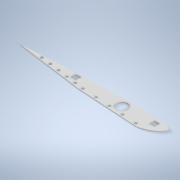
# Autodesk Inventor part: airfoil
Saved by Autodesk Inventor 2021 (Build 250183000, 183)
## iProperties
Created: 2021-03-04
Part Number: airfoil
Material: Generic
Document SubType Name: Modeling
Designer: Ferdinand Hubbard
Density: 1 g/cm^3
Appearance: Default
Author: Ferdinand Hubbard
Autodesk Inventor part; units mm, degrees
ref_plane "YZ Plane" through (0, 0, 0) normal (1, 0, 0) x (0, 1, 0)
ref_plane "XZ Plane" through (0, 0, 0) normal (0, 1, 0) x (-1, 0, 0)
ref_plane "XY Plane" through (0, 0, 0) normal (0, 0, 1) x (1, 0, 0)
sketch "Sketch1" plane through (0, 0, 0) normal (0, 1, 0) x (-1, 0, 0)
  circle A0 centre (105.5716, 8.1262) radius 14.25
  circle A1 centre (105.5716, 8.1262) radius 9.25
  line L0 (22.2, 11.4019) -> (35.2, 11.4019)
  line L1 (35.2, 11.4019) -> (35.2, -1.5981)
  line L2 (35.2, -1.5981) -> (22.2, -1.5981)
  line L3 (22.2, -1.5981) -> (22.2, 11.4019)
  line L4 (218.3762, 9.117) -> (231.3762, 9.117)
  line L5 (231.3762, 9.117) -> (231.3762, -3.883)
  line L6 (231.3762, -3.883) -> (218.3762, -3.883)
  line L7 (218.3762, -3.883) -> (218.3762, 9.117)
  circle A2 centre (364, -0.1617) radius 156.5 construction
  circle A3 centre (201.1292, 22.785) radius 156.5 construction
  line L8 (45.2771, 32.5319) -> (201.1292, 22.785)
  line L9 (363.0659, -0.0318) -> (208.9905, 21.3865)
  circle A4 centre (53.4178, 26.5131) radius 3.5
  circle A5 centre (88.1392, 24.3452) radius 3.5
  circle A6 centre (122.8606, 22.1774) radius 3.5
  circle A7 centre (157.582, 20.0096) radius 3.5
  circle A8 centre (192.3034, 17.8418) radius 3.5
  circle A9 centre (308.9407, 1.9393) radius 3.5
  line L10 (244.7644, 10.8606) -> (145.7169, 24.6294) construction
  line L11 (244.7644, 10.8606) -> (343.8179, -2.909) construction
  line L12 (208.9905, 21.3865) -> (214.4381, 20.6292) construction
  line L13 (308.9407, 1.9393) -> (309.698, 7.387) construction
  line L14 (214.4381, 20.6292) -> (238.2531, 17.3187) construction
  line L15 (238.2531, 17.3187) -> (262.0681, 14.0081) construction
  line L16 (262.0681, 14.0081) -> (285.8831, 10.6975) construction
  line L17 (285.8831, 10.6975) -> (309.6981, 7.3869) construction
  line L18 (214.4381, 20.6292) -> (213.6809, 15.1816) construction
  line L19 (238.2531, 17.3187) -> (237.4959, 11.871) construction
  circle A10 centre (213.6809, 15.1816) radius 3.5
  circle A11 centre (237.4959, 11.871) radius 3.5
  line L20 (262.0681, 14.0081) -> (261.3108, 8.5605) construction
  line L21 (285.8831, 10.6975) -> (285.1258, 5.2499) construction
  circle A12 centre (261.3108, 8.5605) radius 3.5
  circle A13 centre (285.1258, 5.2499) radius 3.5
  spline S0 degree 4 poles (45.2771, 32.5319) (41.5409, 31.6235) (35.6173, 29.7503) (27.9433, 26.9303) (19.3063, 22.5208) (12.8749, 18.2077) (7.7345, 14.0731) (3.8722, 9.2552) (1.4864, 6.2872) (0.043, 1.3745) (-0.0312, 0.3812) (0.0281, -0.8778) (0.1745, -1.4612) (0.3929, -2.0102) (0.8084, -2.4627) (1.3186, -2.8975) (2.6239, -3.7046) (3.653, -4.1929) (10.4393, -6.6384) (15.6655, -7.3545) (25.1, -8.9784) (35.2344, -9.7015) (47.6639, -10.3746) (61.4155, -10.6998) (76.7019, -10.8882) (93.186, -10.8841) (110.736, -10.7454) (129.1149, -10.4736) (148.1138, -10.0951) (167.5031, -9.6193) (187.0543, -9.0657) (206.5356, -8.4416) (225.7153, -7.7631) (244.3709, -7.0324) (262.2765, -6.2607) (279.2509, -5.4328) (295.0539, -4.5223) (309.7119, -3.5525) (322.672, -2.6096) (334.6864, -1.7311) (343.575, -1.0514) (353.0562, -0.487) (356.1651, -0.2567) (362.8735, -0.0152) (362.7416, -0.02) (363.0659, -0.0318) knots 0 0 0 0 0 0.037834 0.062048 0.085007 0.106643 0.126842 0.145458 0.16091 0.173408 0.182937 0.189909 0.196272 0.202293 0.208895 0.216296 0.226837 0.241196 0.259494 0.282121 0.307217 0.334444 0.363559 0.394326 0.426495 0.459817 0.494058 0.528992 0.564399 0.600063 0.635772 0.671312 0.706467 0.741023 0.774768 0.8075 0.839017 0.869102 0.897496 0.923869 0.947785 0.968629 0.984176 1 1 1 1 1
  spline S1 degree 4 poles (208.9905, 21.3865) (207.0256, 21.743) (205.0603, 22.0965) (203.0947, 22.444) (201.1292, 22.785) knots 0.200177 0.200177 0.200177 0.200177 0.200177 0.208976 0.208976 0.208976 0.208976 0.208976
  point P0 (0, 0)
  point P1 (359.0762, 0.1364)
  point P2 (352.983, 0.4477)
  point P3 (344.5923, 1.0476)
  point P4 (334.0615, 2.0094)
  point P5 (321.589, 3.3822)
  point P6 (307.4061, 5.186)
  point P7 (291.7666, 7.4112)
  point P8 (274.9383, 10.0199)
  point P9 (257.194, 12.9452)
  point P10 (238.8043, 16.1074)
  point P11 (220.0304, 19.3803)
  point P12 (182.3116, 25.884)
  point P13 (163.8086, 28.8383)
  point P14 (145.8054, 31.4519)
  point P15 (128.4709, 33.6056)
  point P16 (111.9535, 35.2083)
  point P17 (96.3823, 36.1751)
  point P18 (81.868, 36.4427)
  point P19 (68.5109, 35.9373)
  point P20 (56.3246, 34.585)
  point P21 (26.5856, 26.0467)
  point P22 (18.9844, 22.098)
  point P23 (12.6078, 17.8447)
  point P24 (7.5002, 13.4274)
  point P25 (3.6892, 9.0035)
  point P26 (1.1921, 4.7745)
  point P27 (0.0659, 1.0017)
  point P28 (0.0006, -0.063)
  point P29 (0.0749, -0.9695)
  point P30 (0.2078, -1.5106)
  point P31 (0.424, -1.9791)
  point P32 (0.7616, -2.3945)
  point P33 (1.2282, -2.7955)
  point P34 (2.1216, -3.3822)
  point P35 (3.2232, -3.9537)
  point P36 (8.1428, -5.7128)
  point P37 (15.1176, -7.3056)
  point P38 (23.9224, -8.6283)
  point P39 (34.4841, -9.6094)
  point P40 (46.7728, -10.2571)
  point P41 (60.6811, -10.6511)
  point P42 (76.0314, -10.8426)
  point P43 (92.6351, -10.8589)
  point P44 (110.2911, -10.7246)
  point P45 (128.7881, -10.4591)
  point P46 (147.9055, -10.0812)
  point P47 (167.4164, -9.6062)
  point P48 (187.0898, -9.0495)
  point P49 (206.6927, -8.4228)
  point P50 (225.993, -7.7378)
  point P51 (244.7618, -7.0012)
  point P52 (262.7756, -6.217)
  point P53 (279.8246, -5.3721)
  point P54 (295.7441, -4.4524)
  point P55 (310.4019, -3.4858)
  point P56 (323.6531, -2.5368)
  point P57 (335.3351, -1.6764)
  point P58 (345.271, -0.9701)
  point P59 (353.2753, -0.4606)
  point P60 (359.1655, -0.1576)
  point P61 (362.7814, -0.0252)
  dimension "d2" = 28.5
  dimension "d3" = 18.5
  dimension "d12" = 13
  dimension "d13" = 13
  dimension "d14" = 13
  dimension "d15" = 13
  dimension "d44" = 7
  dimension "d45" = 7
  dimension "d48" = 7
  dimension "d49" = 47.3016
  dimension "d50" = 7
  dimension "d62" = 5.5
  dimension "d71" = 156.1566
  dimension "d72" = 155.557
  constraints: 44 end point, 13 centre point, 11 point on line, 6 coincident, 5 perpendicular, 4 parallel, 2 horizontal, 49 other
  measures "d2" diameter of A0
  measures "d3" diameter of A1
  measures "d12" distance of L1.end L2.end
  measures "d13" distance of L0.end L1.end
  measures "d14" distance of L5.end L6.end
  measures "d15" distance of L4.end L5.end
  measures "d44" diameter of A4
  measures "d45" diameter of A5
  measures "d48" diameter of A8
  measures "d49" vertical distance of point (92.635, -10.859) point (81.868, 36.443)
  measures "d50" diameter of A9
  measures "d62" distance of L12.end L18.end
  measures "d71" distance of L8.start L8.end
  measures "d72" distance of L9.end L9.start
extrude "Extrusion1" add sketch "Sketch1" along normal blind 2 contours L8 S1 L9 S0
body "Solid1"
